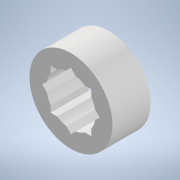
# Autodesk Inventor part: oponka
Saved by Autodesk Inventor 2022.3 (Build 263350000, 350)
## iProperties
Created: 2022-12-14
Part Number: oponka
Material: Generic
Document SubType Name: Modeling
Designer: komputer
Density: 1 g/cm^3
Appearance: Default
Author: komputer
Autodesk Inventor part; units mm, degrees
ref_plane "YZ Plane" through (0, 0, 0) normal (1, 0, 0) x (0, 1, 0)
ref_plane "XZ Plane" through (0, 0, 0) normal (0, 1, 0) x (-1, 0, 0)
sketch "Sketch1" plane through (0, 0, 0) normal (0, 0, 1) x (1, 0, 0)
  line L0 (-2.3998, 1.6282) -> (-2.4042, 2.4042) projected
  arc A0 (-2.3998, 1.6282) -> (-2.8482, 0.5456) centre (0, 0) ccw projected
  line L1 (-3.4, 0) -> (-2.8482, 0.5456) projected
  line L2 (-2.8482, -0.5456) -> (-3.4, 0) projected
  arc A1 (-2.8482, -0.5456) -> (-2.3998, -1.6282) centre (0, 0) ccw projected
  line L3 (-2.4042, -2.4042) -> (-2.3998, -1.6282) projected
  line L4 (-1.6282, -2.3998) -> (-2.4042, -2.4042) projected
  arc A2 (-1.6282, -2.3998) -> (-0.5456, -2.8482) centre (0, 0) ccw projected
  line L5 (0, -3.4) -> (-0.5456, -2.8482) projected
  line L6 (0.5456, -2.8482) -> (0, -3.4) projected
  arc A3 (0.5456, -2.8482) -> (1.6282, -2.3998) centre (0, 0) ccw projected
  line L7 (2.4042, -2.4042) -> (1.6282, -2.3998) projected
  line L8 (2.3998, -1.6282) -> (2.4042, -2.4042) projected
  arc A4 (2.3998, -1.6282) -> (2.8482, -0.5456) centre (0, 0) ccw projected
  line L9 (3.4, 0) -> (2.8482, -0.5456) projected
  line L10 (2.8482, 0.5456) -> (3.4, 0) projected
  arc A5 (2.8482, 0.5456) -> (2.3998, 1.6282) centre (0, 0) ccw projected
  line L11 (2.4042, 2.4042) -> (2.3998, 1.6282) projected
  line L12 (1.6282, 2.3998) -> (2.4042, 2.4042) projected
  arc A6 (1.6282, 2.3998) -> (0.5456, 2.8482) centre (0, 0) ccw projected
  line L13 (0, 3.4) -> (0.5456, 2.8482) projected
  line L14 (-0.5456, 2.8482) -> (0, 3.4) projected
  arc A7 (-0.5456, 2.8482) -> (-1.6282, 2.3998) centre (0, 0) ccw projected
  line L15 (-2.4042, 2.4042) -> (-1.6282, 2.3998) projected
  circle A8 centre (0, 0) radius 1 projected
  circle A9 centre (0, 0) radius 2.9
  circle A10 centre (0, 0) radius 1.1 projected
  line L16 (-12.5394, 7.938) -> (-12.4815, -3.7618) projected
  line L17 (-12.4815, -3.7618) -> (12.5182, -3.6381) projected
  line L18 (12.5182, -3.6381) -> (12.4603, 8.0618) projected
  line L19 (12.4603, 8.0618) -> (-12.5394, 7.938) projected
  circle A11 centre (8.485, 3.042) radius 3 projected
  circle A12 centre (-8.5147, 2.9579) radius 3 projected
  line L20 (0, 0) -> (0.0183, -3.7)
  line L21 (0.0183, -3.7) -> (0.0243, -4.8999)
  circle A13 centre (0, 0) radius 4.9
  point P0 (0, 0)
  dimension "d0" = 1.2
  constraints: 4 end point, 2 coincident, 1 centre point, 1 midpoint, 1 point on line, 3 other
  measures "d0" distance of L20.end L21.end
ref_plane "Work Plane1" through (-3.4, -3.4, -4.5) normal (0, 0, -1) x (0, 1, 0)
extrude "Extrusion1" add sketch "Sketch1" against normal up to surface (4.5 mm away) contours L17 A13 | L17 A13 L21 | L21 A13 L17
body "Solid1"
